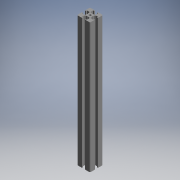
# Autodesk Inventor part: HFS3-1515-150
Saved by Autodesk Inventor 2017.3 (Build 213256000, 256)
## iProperties
Part Number: HFS3-1515-150
Material: Generic
Catalog Web Link: www.cadenas.de
Description: HFS3, KHFS3-Aluminum Frames 15mm Square
Vendor: MISUMI
Document SubType Name: Modeling
Designer: partserver
Manufacturer: MISUMI
Mass: 18.8122 g
Surface Area: 178.104 cm^2
Volume: 18.8122 cm^3
Density: 1 g/cm^3
Appearance: PSOLRGB-175-175-175
Category: PARTsolutions
Company: MISUMI
Title: HFS3-1515-150
Author: Cadenas PARTsolutions
Comments: Aluminum Frames 15mm Square
L: 150
PSOL_IDENT_0: {$CADENAS_DATA\23d-libs\misumi\metric\38_al_extrusions_blackets\hfs3_1515.prj},173 {VTYP=3D},{NB=HFS
PSOL_IDENT_1: 3-1515-150},{LINA=HFS3-1515-150},{NN=HFS3, KHFS3},{DATE=08.06.2021 08:27:33},{GEOMDATE=07.03.2008 00
PSOL_IDENT_2: :00:00},{VERSION=},{LINEID=10},{WBVAR=L},{WBNUMERIC=L}  {NB=HFS3-1515-150},{LINA=HFS3-1515-150},{KT=
PSOL_IDENT_3: LINA},{PN=HFS3-1515-150},{MAT=A6N01SS-T5(Aluminum)(EN AC-51400_AlMgSiO,7-T5)},{ST=Alumite},{LT=Speci
PSOL_IDENT_4: fied Length},{L=150.0},{FEAT=4 Slots},{LALG=[50-2000/0.5]},{LTOL=+/- 0.5},{MASS=0.34},{SA=126},{SMIL
PSOL_IDENT_5: X=0.280x10^4},{SMILY=0.280x10^4},{TYPE=HFS3-1515}
NB: HFS3-1515-150
NN: HFS3, KHFS3
NT: Aluminum Frames 15mm Square
NBSYN: $PN.
LINA: HFS3-1515-150
CATALOG: Misumi
PN: HFS3-1515-150
MAT: A6N01SS-T5
ST: Clear Anodizing
LT: Specified Length
LTOL: +/- 0.5
MASS: 0.34
SA: 126
SMILX: 0.280x10^4
SMILY: 0.280x10^4
SUPPLIER: MISUMI
ARTICLENO: HFS3-1515-150
BOMINFO: HFS3-1515-150
CREATOR: CADENAS GmbH
Autodesk Inventor part; units mm, degrees
ref_plane "YZ Plane" through (0, 0, 0) normal (1, 0, 0) x (0, 1, 0)
ref_plane "XZ Plane" through (0, 0, 0) normal (0, 1, 0) x (-1, 0, 0)
ref_plane "XY Plane" through (0, 0, 0) normal (0, 0, 1) x (1, 0, 0)
sketch "Sketch_1" plane through (0, 0, 0) normal (0, 0, 1) x (1, 0, 0)
  arc A0 (-7.5, 2) -> (-7.2, 1.7) centre (-7.2, 2) ccw
  line L0 (-7.2, 1.7) -> (-6.4, 1.7)
  line L1 (-6.4, 1.7) -> (-6.4, 2.85)
  line L2 (-6.4, 2.85) -> (-3.8, 2.85)
  line L3 (-3.8, 2.85) -> (-2.8, 1.85)
  line L4 (-2.8, 1.85) -> (-2.8, 0.5196)
  line L5 (-2.8, 0.5196) -> (-2.5, 0)
  line L6 (-2.5, 0) -> (-2.8, -0.5196)
  line L7 (-2.8, -0.5196) -> (-2.8, -1.85)
  line L8 (-2.8, -1.85) -> (-3.8, -2.85)
  line L9 (-3.8, -2.85) -> (-6.4, -2.85)
  line L10 (-6.4, -2.85) -> (-6.4, -1.7)
  line L11 (-6.4, -1.7) -> (-7.2, -1.7)
  arc A1 (-7.2, -1.7) -> (-7.5, -2) centre (-7.2, -2) ccw
  line L12 (-7.5, -2) -> (-7.5, -6.5)
  arc A2 (-7.5, -6.5) -> (-6.5, -7.5) centre (-6.5, -6.5) ccw
  line L13 (-6.5, -7.5) -> (-2, -7.5)
  arc A3 (-2, -7.5) -> (-1.7, -7.2) centre (-2, -7.2) ccw
  line L14 (-1.7, -7.2) -> (-1.7, -6.4)
  line L15 (-1.7, -6.4) -> (-2.85, -6.4)
  line L16 (-2.85, -6.4) -> (-2.85, -3.8)
  line L17 (-2.85, -3.8) -> (-1.85, -2.8)
  line L18 (-1.85, -2.8) -> (-0.5196, -2.8)
  line L19 (-0.5196, -2.8) -> (0, -2.5)
  line L20 (0, -2.5) -> (0.5196, -2.8)
  line L21 (0.5196, -2.8) -> (1.85, -2.8)
  line L22 (1.85, -2.8) -> (2.85, -3.8)
  line L23 (2.85, -3.8) -> (2.85, -6.4)
  line L24 (2.85, -6.4) -> (1.7, -6.4)
  line L25 (1.7, -6.4) -> (1.7, -7.2)
  arc A4 (1.7, -7.2) -> (2, -7.5) centre (2, -7.2) ccw
  line L26 (2, -7.5) -> (6.5, -7.5)
  arc A5 (6.5, -7.5) -> (7.5, -6.5) centre (6.5, -6.5) ccw
  line L27 (7.5, -6.5) -> (7.5, -2)
  arc A6 (7.5, -2) -> (7.2, -1.7) centre (7.2, -2) ccw
  line L28 (7.2, -1.7) -> (6.4, -1.7)
  line L29 (6.4, -1.7) -> (6.4, -2.85)
  line L30 (6.4, -2.85) -> (3.8, -2.85)
  line L31 (3.8, -2.85) -> (2.8, -1.85)
  line L32 (2.8, -1.85) -> (2.8, -0.5196)
  line L33 (2.8, -0.5196) -> (2.5, 0)
  line L34 (2.5, 0) -> (2.8, 0.5196)
  line L35 (2.8, 0.5196) -> (2.8, 1.85)
  line L36 (2.8, 1.85) -> (3.8, 2.85)
  line L37 (3.8, 2.85) -> (6.4, 2.85)
  line L38 (6.4, 2.85) -> (6.4, 1.7)
  line L39 (6.4, 1.7) -> (7.2, 1.7)
  arc A7 (7.2, 1.7) -> (7.5, 2) centre (7.2, 2) ccw
  line L40 (7.5, 2) -> (7.5, 6.5)
  arc A8 (7.5, 6.5) -> (6.5, 7.5) centre (6.5, 6.5) ccw
  line L41 (6.5, 7.5) -> (2, 7.5)
  arc A9 (2, 7.5) -> (1.7, 7.2) centre (2, 7.2) ccw
  line L42 (1.7, 7.2) -> (1.7, 6.4)
  line L43 (1.7, 6.4) -> (2.85, 6.4)
  line L44 (2.85, 6.4) -> (2.85, 3.8)
  line L45 (2.85, 3.8) -> (1.85, 2.8)
  line L46 (1.85, 2.8) -> (0.5196, 2.8)
  line L47 (0.5196, 2.8) -> (0, 2.5)
  line L48 (0, 2.5) -> (-0.5196, 2.8)
  line L49 (-0.5196, 2.8) -> (-1.85, 2.8)
  line L50 (-1.85, 2.8) -> (-2.85, 3.8)
  line L51 (-2.85, 3.8) -> (-2.85, 6.4)
  line L52 (-2.85, 6.4) -> (-1.7, 6.4)
  line L53 (-1.7, 6.4) -> (-1.7, 7.2)
  arc A10 (-1.7, 7.2) -> (-2, 7.5) centre (-2, 7.2) ccw
  line L54 (-2, 7.5) -> (-6.5, 7.5)
  arc A11 (-6.5, 7.5) -> (-7.5, 6.5) centre (-6.5, 6.5) ccw
  line L55 (-7.5, 6.5) -> (-7.5, 2)
  circle A12 centre (0, 0) radius 1.25
  constraints: 112 end point, 24 point on circle, 13 centre point
extrude "Extrusion1" add sketch "Sketch_1" along normal blind 150
equation "\"d0\" = L"
equation "\"L\" = 150"
body "Solid1"
